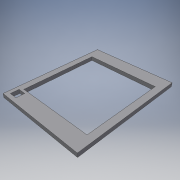
# Autodesk Inventor part: monitor frame part1 (for assembly)
Saved by Autodesk Inventor 2016 (Build 200138000, 138)
## iProperties
Created: 2017-10-23
Part Number: monitor frame part1 (for assembly)
Material: Generic
Document SubType Name: Modeling
Designer: student
Density: 1 g/cm^3
Appearance: Default
Author: student
Autodesk Inventor part; units mm, degrees
ref_plane "YZ Plane" through (0, 0, 0) normal (1, 0, 0) x (0, 1, 0)
ref_plane "XZ Plane" through (0, 0, 0) normal (0, 1, 0) x (-1, 0, 0)
ref_plane "XY Plane" through (0, 0, 0) normal (0, 0, 1) x (1, 0, 0)
sketch "Sketch1" plane through (0, 0, 0) normal (0, 1, 0) x (-1, 0, 0)
  line L0 (-203.2, 254) -> (203.2, 254)
  line L1 (203.2, 254) -> (203.2, -254)
  line L2 (203.2, -254) -> (-203.2, -254)
  line L3 (-203.2, -254) -> (-203.2, 254)
  line L4 (-203.2, 254) -> (203.2, -254) construction
  line L5 (203.2, 254) -> (-203.2, -254) construction
  point P0 (0, 0)
  dimension "d0" = 508
  dimension "d1" = 406.4
  constraints: 12 end point, 2 midpoint, 2 parallel, 1 horizontal, 1 perpendicular
  measures "d0" distance of L0.end L1.end
  measures "d1" distance of L1.end L2.end
extrude "Extrusion1" add sketch "Sketch1" along normal blind 19.05
sketch "Sketch2" plane through (0, 19.05, 0) normal (0, 1, 0) x (1, 0, 0)
  line L0 (171.45, -184.15) -> (-171.45, -184.15)
  line L1 (-171.45, -184.15) -> (-171.45, 184.15)
  line L2 (-171.45, 184.15) -> (171.45, 184.15)
  line L3 (171.45, 184.15) -> (171.45, -184.15)
  line L4 (171.45, -184.15) -> (-171.45, 184.15) construction
  line L5 (-171.45, -184.15) -> (171.45, 184.15) construction
  point P0 (0, 0)
  dimension "d4" = 368.3
  dimension "d5" = 342.9
  constraints: 12 end point, 2 midpoint, 2 parallel, 1 horizontal, 1 perpendicular
  measures "d4" distance of L0.end L1.end
  measures "d5" distance of L1.end L2.end
extrude "Extrusion2" cut sketch "Sketch2" against normal blind 25.4
sketch "Sketch3" plane through (0, 19.05, 0) normal (0, 1, 0) x (1, 0, 0)
  line L0 (-184.15, -196.85) -> (-184.15, -234.95)
  line L1 (-184.15, -234.95) -> (-146.05, -234.95)
  line L2 (-146.05, -234.95) -> (-146.05, -196.85)
  line L3 (-203.2, 254) -> (-203.2, -254) projected
  line L4 (-146.05, -196.85) -> (-184.15, -196.85)
  line L5 (-203.2, -254) -> (203.2, -254) projected
  point P0 (0, 0)
  dimension "d9" = 19.05
  dimension "d10" = 38.1
  dimension "d13" = 38.1
  dimension "d14" = 19.05
  constraints: 8 end point, 3 perpendicular
  measures "d9" distance between parallel lines of L3 L0
  measures "d10" distance between parallel lines of L0 L2
  measures "d13" distance between parallel lines of L1 L4
  measures "d14" distance between parallel lines of L5 L1
extrude "Extrusion3" cut sketch "Sketch3" against normal blind 25.4
body "Solid1"
